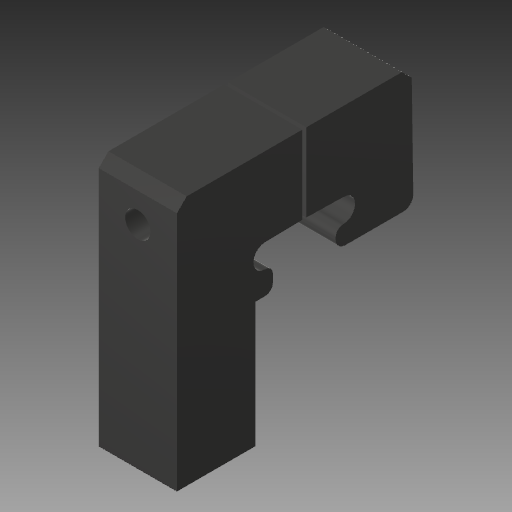
# Autodesk Inventor part: Corner Clamp
Saved by Autodesk Inventor 2019 (Build 230136000, 136)
## iProperties
Created: 2020-12-25
Part Number: Corner Clamp
Material: Acetal Resin, Black
Document SubType Name: Modeling
Designer: John
Density: 1.425 g/cm^3
Appearance: Smooth - Black
Author: John
Autodesk Inventor part; units mm, degrees
ref_plane "YZ Plane" through (0, 0, 0) normal (1, 0, 0) x (0, 1, 0)
ref_plane "XZ Plane" through (0, 0, 0) normal (0, 1, 0) x (-1, 0, 0)
ref_plane "XY Plane" through (0, 0, 0) normal (0, 0, 1) x (1, 0, 0)
sketch "Sketch1" plane through (0, 0, 0) normal (1, 0, 0) x (0, 1, 0)
  line L0 (-3.175, -15.8752) -> (-3.175, 15.8752)
  arc A0 (18.3756, 12.6998) -> (12.0256, 12.7) centre (15.2006, 12.6998) ccw
  arc A1 (12.0256, -12.7002) -> (18.3756, -12.7002) centre (15.2006, -12.7002) ccw
  line L1 (8.8506, 9.5252) -> (6.35, 9.5252)
  line L2 (8.8506, -9.5252) -> (5.1346, -9.5252)
  line L3 (15.2006, 12.6998) -> (15.2006, -12.7002) construction
  line L4 (3.175, 14.6052) -> (3.175, 12.7002)
  arc A2 (8.8506, 9.5252) -> (12.0256, 12.7) centre (8.8506, 12.7002) ccw
  arc A3 (12.0256, -12.7002) -> (8.8506, -9.5252) centre (8.8506, -12.7002) ccw
  arc A4 (3.175, 12.7002) -> (6.35, 9.5252) centre (6.35, 12.7002) ccw
  arc A5 (5.1346, -9.5252) -> (1.9937, -12.2364) centre (5.1346, -12.7002) ccw
  line L5 (-3.175, -15.8752) -> (-3.175, -22.2252)
  line L6 (1.905, 15.8752) -> (-3.175, 15.8752)
  arc A6 (3.175, 14.6052) -> (1.905, 15.8752) centre (1.905, 14.6052) ccw
  line L7 (18.3756, 12.6998) -> (18.3756, -12.7002)
  line L8 (1.6475, -13.2791) -> (-3.175, -22.2252)
  arc A7 (1.6475, -13.2791) -> (1.9937, -12.2364) centre (-1.1473, -11.7726) ccw
  line L9 (44.6375, 0.635) -> (19.2375, 0.635)
  line L10 (19.2375, 0.635) -> (19.2375, -0.635) construction
  line L11 (19.2375, -0.635) -> (44.6375, -0.635)
  line L12 (44.6375, -0.635) -> (44.6375, 0.635) construction
  line L13 (44.6375, 0.635) -> (19.2375, -0.635) construction
  line L14 (19.2375, 0.635) -> (44.6375, -0.635) construction
  line L15 (-13.1873, 0) -> (54.275, 0) projected
  line L16 (44.6375, -0.635) -> (44.6375, -26.035)
  line L17 (35.6573, -35.0153) -> (8.3561, -35.4163)
  line L18 (5.1346, -32.2418) -> (5.1346, -13.3352)
  line L19 (44.6375, 0.635) -> (44.6375, 32.385)
  line L20 (35.6573, 41.3653) -> (3.81, 41.3653)
  arc A8 (5.1346, -32.2418) -> (8.3561, -35.4163) centre (8.3094, -32.2418) ccw
  arc A9 (8.8506, 10.1602) -> (11.3906, 12.7) centre (8.8506, 12.7002) ccw
  line L21 (8.8506, 10.1602) -> (6.35, 10.1602)
  arc A10 (3.81, 12.7002) -> (6.35, 10.1602) centre (6.35, 12.7002) ccw
  line L22 (3.81, 12.7002) -> (3.81, 41.3653)
  line L23 (8.3096, -10.1602) -> (8.8506, -10.1602)
  arc A11 (11.3906, -12.7002) -> (8.8506, -10.1602) centre (8.8506, -12.7002) ccw
  arc A12 (11.3906, -12.7002) -> (19.0106, -12.7002) centre (15.2006, -12.7002) ccw
  arc A13 (19.0106, 12.6998) -> (11.3906, 12.7) centre (15.2006, 12.6998) ccw
  line L24 (-3.5499, 0) -> (-3.5499, -1.7744)
  line L25 (19.0106, -12.7002) -> (19.2375, -0.635)
  line L26 (19.2375, 0.635) -> (19.0106, 12.6998)
  arc A14 (8.3096, -10.1602) -> (5.1346, -13.3352) centre (8.3096, -13.3352) ccw
  line L27 (-3.175, -22.2252) -> (1.6475, -22.2252)
  line L28 (35.6573, 41.3653) -> (44.6375, 41.3653)
  line L29 (44.6375, 41.3653) -> (44.6375, 32.385)
  line L30 (44.6375, -26.035) -> (44.6375, -34.8834)
  line L31 (44.6375, -34.8834) -> (35.6573, -35.0153)
  point P0 (0, 0)
  point P1 (15.2516, 9.5252)
  point P2 (15.2006, -9.5252)
  point P3 (1.9596, -12.7002)
  point P4 (31.9375, 0)
  point P5 (31.9375, 0)
  dimension "d5" = 6.35
  dimension "d8" = 3.175
  dimension "d9" = 6.35
  dimension "d11" = 6.35
  dimension "d12" = 6.35
  dimension "d13" = 1.27
  dimension "d30" = 25.4
  dimension "d31" = 3.175
  dimension "d51" = 1.27
  dimension "d54" = 25.4
  dimension "d56" = 25.4
  dimension "d59" = 31.75
  dimension "d60" = 0.635
  dimension "d61" = 3.175
  constraints: 62 end point, 33 point on circle, 17 tangent, 15 centre point, 8 vertical, 7 perpendicular, 6 parallel, 6 point on line, 4 equal radius, 4 horizontal, 3 midpoint, 2 collinear, 6 other
  measures "d5" diameter of A1
  measures "d8" radius of A2
  measures "d9" distance of L0.start L5.end
  measures "d11" distance between parallel lines of L1 L6
  measures "d12" distance from line of L0.start L2
  measures "d13" radius of A6
  measures "d30" distance of L3.start L3.end
  measures "d31" radius of A7
  measures "d51" distance of L11.end L9.start
  measures "d54" distance of L10.end L11.end
  measures "d56" distance of L11.end L16.end
  measures "d59" distance of L9.start L19.end
  measures "d60" radial gap between concentric circles of A0 A13
  measures "d61" radius of A14
extrude "Extrusion8" add sketch "Sketch1" along normal mid plane 25.4 contours L9 L26 A13 A9 L21 A10 L22 L20 L28 L29 L19 | L11 L16 L30 L31 L17 A8 L18 A14 L23 A11 A12 L25
sketch "Sketch8" plane through (-12.7, 3.81, 12.7002) normal (0, -1, 0) x (1, 0, 0)
  line L0 (25.4, 28.6651) -> (0, 28.6651) projected
  line L1 (0, 28.6651) -> (25.4, 28.6651)
  line L2 (25.4, 28.6651) -> (25.4, 3.1762)
  line L3 (25.4, 3.1762) -> (0, 3.1762)
  line L4 (0, 3.1762) -> (0, 28.6651)
  point P0 (12.7, -12.7002)
  dimension "d83" = 25.4889
  constraints: 8 end point, 2 parallel, 1 horizontal, 1 perpendicular
  measures "d83" distance of L1.end L2.end
ref_plane "Work Plane12" through (-12.7, 35.6573, 41.3653) normal (0, 0, 1) x (1, 0, 0)
sketch "Sketch9" plane through (-12.7, 35.6573, 41.3653) normal (0, 0, 1) x (1, 0, 0)
  line L0 (0, -16.4197) -> (25.4, -16.4197) projected
  line L1 (25.4, 8.9803) -> (25.4, -16.4197) projected
  line L2 (25.4, 8.9803) -> (0, 8.9803) projected
  line L3 (0, -16.4197) -> (0, 8.9803) projected
  circle A0 centre (12.7, -3.7197) radius 2.2225
  point P0 (12.7, -35.6573)
  dimension "d68" = 4.445
  constraints: 1 centre point
  measures "d68" diameter of A0
extrude "Extrusion10" cut sketch "Sketch9" against normal through all contours A0
ref_plane "Work Plane13" through (-12.7, 35.6573, 41.3653) normal (0, 0, 1) x (1, 0, 0)
sketch "Sketch10" plane through (-12.7, 35.6573, 41.3653) normal (0, 0, 1) x (1, 0, 0)
  circle A0 centre (12.7, -3.7197) radius 2.2225 projected
  circle A1 centre (12.7, -3.7197) radius 4.1275
  point P0 (12.7, -35.6573)
  dimension "d71" = 8.255
  constraints: 1 centre point, 1 coincident
  measures "d71" diameter of A1
extrude "Extrusion11" cut sketch "Sketch10" against normal blind 34.925
sketch "Sketch11" plane through (12.7, 35.6573, -35.0153) normal (0, 0.0146866, -0.9998921) x (-1, 0, 0)
  ellipse E0 centre (12.7, -3.7201) end of major axis (12.7, -1.4974) minor radius 2.2225 projected
  circle A0 centre (12.7, -3.7201) radius 6.35
  point P0 (12.7, -35.1392)
  dimension "d74" = 12.7
  constraints: 1 centre point, 1 coincident, 1 other
  measures "d74" diameter of A0
extrude "Extrusion12" cut sketch "Sketch11" against normal blind 28.575 contours E0 | A0
chamfer "Chamfer1" distance 3.175 angle 45 2 edges at (0, 44.6375, 41.3653) (0, 44.6375, -34.8834)
extrude "Extrusion14" add sketch "Sketch8" along normal blind 40.64
body "Solid3"
